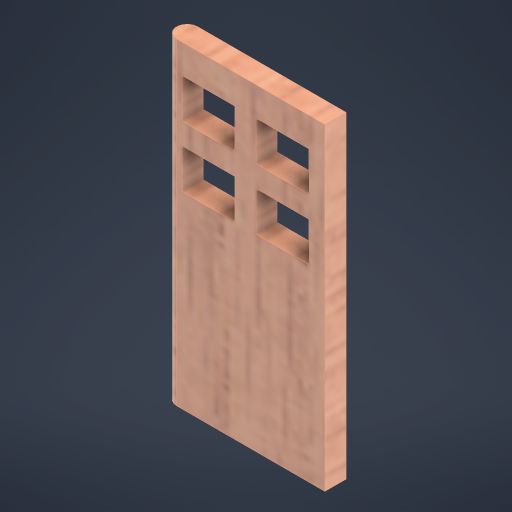
# Autodesk Inventor part: dvere
Saved by Autodesk Inventor 2023 (Build 270158000, 158)
## iProperties
Created: 2022-10-19
Part Number: dvere
Material: Dřevo (dub)
Document SubType Name: Modeling
Designer: zak
Density: 0.76 g/cm^3
Appearance: Dub zimní – přírodní – střední lesk
Mass: 4.42799 g
Surface Area: 42.6781 cm^2
Volume: 5.82631 cm^3
Author: zak
Autodesk Inventor part; units mm, degrees
ref_plane "YZ Plane" through (0, 0, 0) normal (1, 0, 0) x (0, 1, 0)
ref_plane "XZ Plane" through (0, 0, 0) normal (0, 1, 0) x (-1, 0, 0)
ref_plane "XY Plane" through (0, 0, 0) normal (0, 0, 1) x (1, 0, 0)
sketch "Náčrt1" plane through (0, 0, 0) normal (0, 0, 1) x (1, 0, 0)
  line L0 (-15, -30) -> (15, -30)
  line L1 (15, -30) -> (15, 30)
  line L2 (15, 30) -> (-15, 30)
  line L3 (-15, 30) -> (-15, -30)
  line L4 (-15, -30) -> (15, 30) construction
  line L5 (15, -30) -> (-15, 30) construction
  line L6 (0, 30) -> (0, 0)
  line L7 (-15, 15) -> (15, 15)
  line L8 (2, 17) -> (12, 17)
  line L9 (12, 17) -> (12, 24.5)
  line L10 (12, 24.5) -> (2, 24.5)
  line L11 (2, 24.5) -> (2, 17)
  line L12 (-2, 17) -> (-12, 17)
  line L13 (-12, 17) -> (-12, 24.5)
  line L14 (-12, 24.5) -> (-2, 24.5)
  line L15 (-2, 24.5) -> (-2, 17)
  line L16 (2, 13) -> (12, 13)
  line L17 (12, 13) -> (12, 5.5)
  line L18 (12, 5.5) -> (2, 5.5)
  line L19 (2, 5.5) -> (2, 13)
  line L20 (-12, 5.5) -> (-2, 5.5)
  line L21 (-12, 13) -> (-12, 5.5)
  line L22 (-2, 13) -> (-12, 13)
  line L23 (-2, 5.5) -> (-2, 13)
  dimension "d0" = 30
  dimension "d1" = 60
  dimension "d2" = 15
  dimension "d3" = 10
  dimension "d4" = 7.5
  dimension "d5" = 2
  dimension "d6" = 2
  constraints: 48 end point, 12 symmetric about line, 4 parallel, 3 midpoint, 3 perpendicular, 2 horizontal, 2 point on line, 1 vertical
  measures "d0" distance of L2.end L1.end
  measures "d1" distance of L1.end L0.end
  measures "d2" distance between parallel lines of L2 L7
  measures "d3" distance of L10.end L9.end
  measures "d4" distance of L9.end L8.end
  measures "d5" distance between parallel lines of L6 L11
  measures "d6" distance between parallel lines of L7 L8
extrude "Vysunutí1" add sketch "Náčrt1" along normal blind 4
fillet "Zaoblení1" radius 2 2 edges at (-15, 0, 4) (-15, 0, 0)
sketch "Náčrt2" plane through (15, -30, 0) normal (0, -1, 0) x (1, 0, 0)
  arc A0 (-28, 4) -> (-28, 0) centre (-28, 2) ccw projected
  circle A1 centre (-28, 2) radius 1.5
  point P0 (-15, 0)
  dimension "d10" = 3
  constraints: 1 centre point, 1 coincident
  measures "d10" diameter of A1
extrude "Vysunutí2" cut sketch "Náčrt2" against normal blind 10
